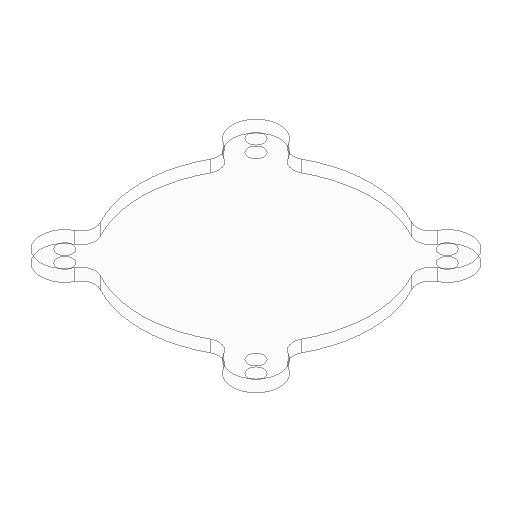
# Autodesk Inventor part: 3DP_ABS_Electronics_Colling_Fan_Grill_Honeycomb
Saved by Autodesk Inventor 2026.1 (Build 301233000, 233)
## iProperties
Created: 2017-07-01
Part Number: 3DP_ABS_Electronics_Colling_Fan_Grill_Honeycomb
Material: Aluminium 5005-H12
Document SubType Name: Modeling
Designer: Andrzej
Density: 2.7 g/cm^3
Appearance: Przezroczyste
Author: Andrzej
Autodesk Inventor part; units mm, degrees
ref_plane "YZ Plane" through (0, 0, 0) normal (1, 0, 0) x (0, 1, 0)
ref_plane "XZ Plane" through (0, 0, 0) normal (0, 1, 0) x (-1, 0, 0)
ref_plane "XY Plane" through (0, 0, 0) normal (0, 0, 1) x (1, 0, 0)
sketch "Szkic1" plane through (0, 0, 0) normal (0, 0, 1) x (1, 0, 0)
  circle A0 centre (-23.62, 45.242) radius 1.65
  circle A1 centre (16.38, 45.242) radius 1.65
  circle A2 centre (-23.62, 5.242) radius 1.65
  circle A3 centre (16.38, 5.242) radius 1.65
  circle A4 centre (-3.62, 25.242) radius 24
  arc A5 (-18.8305, 43.8065) -> (-22.1845, 40.4524) centre (-23.62, 45.242) ccw
  arc A6 (-22.1845, 10.0315) -> (-18.8305, 6.6774) centre (-23.62, 5.242) ccw
  arc A7 (14.9445, 40.4524) -> (11.5905, 43.8065) centre (16.38, 45.242) ccw
  arc A8 (11.5905, 6.6774) -> (14.9445, 10.0315) centre (16.38, 5.242) ccw
  point P0 (0, 0)
  point P1 (0, 0)
  dimension "d10" = 3.3
  dimension "d11" = 3.3
  dimension "d12" = 3.3
  dimension "d15" = 10
  dimension "d16" = 10
  dimension "d17" = 10
  dimension "d18" = 10
  dimension "d22" = 3.3
  constraints: 9 coincident, 8 centre point, 8 point on circle, 10 other
  measures "d10" diameter of A0
  measures "d11" diameter of A1
  measures "d12" diameter of A2
  measures "d15" diameter of A5
  measures "d16" diameter of A6
  measures "d17" diameter of A7
  measures "d18" diameter of A8
  measures "d22" diameter of A3
extrude "Wyciągnięcie proste1" add sketch "Szkic1" along normal blind 2.5
fillet "Zaokrąglenie1" radius 3 8 edges at (-22.1845, 10.0315, 1.25) (-18.8305, 6.6774, 1.25) (14.9445, 10.0315, 1.25) (11.5905, 6.6774, 1.25) (11.5905, 43.8065, 1.25) (14.9445, 40.4524, 1.25) (-18.8305, 43.8065, 1.25) (-22.1845, 40.4524, 1.25)
equation "\"d10\" = d12"
equation "\"d11\" = d12"
equation "\"d22\" = d12"
